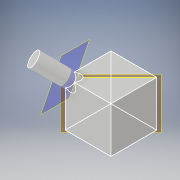
# Autodesk Inventor part: cube
Saved by Autodesk Inventor 2019 (Build 230136000, 136)
## iProperties
Created: 2018-09-07
Part Number: cube
Material: Generic
Document SubType Name: Modeling
Designer: HIVE
Density: 1 g/cm^3
Appearance: Default
Author: HIVE
Autodesk Inventor part; units mm, degrees
ref_plane "YZ Plane" through (0, 0, 0) normal (1, 0, 0) x (0, 1, 0)
ref_plane "XZ Plane" through (0, 0, 0) normal (0, 1, 0) x (-1, 0, 0)
ref_plane "XY Plane" through (0, 0, 0) normal (0, 0, 1) x (1, 0, 0)
sketch "Sketch1" plane through (0, 0, 0) normal (0, 1, 0) x (-1, 0, 0)
  line L0 (-12.5, -12.5) -> (12.5, -12.5)
  line L1 (12.5, -12.5) -> (12.5, 12.5)
  line L2 (12.5, 12.5) -> (-12.5, 12.5)
  line L3 (-12.5, 12.5) -> (-12.5, -12.5)
  line L4 (-12.5, -12.5) -> (12.5, 12.5) construction
  line L5 (12.5, -12.5) -> (-12.5, 12.5) construction
  point P0 (0, 0)
  dimension "d0" = 25
  dimension "d1" = 25
  constraints: 12 end point, 2 midpoint, 2 parallel, 1 horizontal, 1 perpendicular
  measures "d0" distance of L2.end L1.end
  measures "d1" distance of L0.end L1.end
extrude "Extrusion1" add sketch "Sketch1" along normal mid plane 25
ref_plane "Work Plane2" through (-12.5, 12.5, 12.5) normal (0.7071068, 0, 0.7071068) x (0, -1, 0)
ref_plane "Work Plane1" through (12.5, -12.5, -12.5) normal (0.7071068, 0, 0.7071068) x (0, -1, 0)
sketch "Sketch2" plane through (-12.5, 12.5, 12.5) normal (0.7071068, 0, 0.7071068) x (0, -1, 0)
  line L0 (25, 17.6777) -> (25, 35.3553) projected
  line L1 (25, 35.3553) -> (25, 17.6777) projected
  line L2 (25, 17.6777) -> (25, 0) projected
  line L3 (25, 0) -> (25, 17.6777) projected
  line L4 (0, 35.3553) -> (0, 17.6777) projected
  line L5 (0, 17.6777) -> (0, 0) projected
  line L6 (0, 0) -> (0, 17.6777) projected
  line L7 (0, 17.6777) -> (0, 35.3553) projected
  line L8 (0, 0) -> (0, 17.6777) projected
  line L9 (25, 35.3553) -> (25, 17.6777) projected
  line L10 (0, 0) -> (25, 35.3553)
  point P0 (12.5, 17.6777)
  constraints: 2 end point
ref_plane "Work Plane3" through (-12.5, 12.5, 12.5) normal (0.5773503, -0.5773503, -0.5773503) x (0.7071068, 0.7071068, 0)
sketch "Sketch3" plane through (-12.5, 12.5, 12.5) normal (0.5773503, -0.5773503, -0.5773503) x (0.7071068, 0.7071068, 0)
  circle A0 centre (0, 0) radius 4
  dimension "d4" = 8
  constraints: 1 centre point, 1 coincident
  measures "d4" diameter of A0
extrude "Extrusion2" add sketch "Sketch3" along normal blind 10 and the other way blind 15
body "Solid1"
